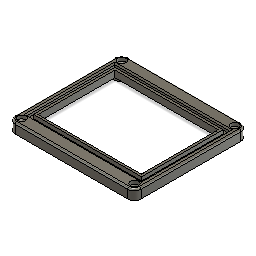
RPLIDAR Enclosure Lid (Bottom) v4 (Autodesk Fusion 360 design; units mm, degrees)
Autodesk Fusion 360 part; units mm, degrees
note: some values were not read from the file. Set by a fixed rule: which sketch regions a step uses.
sketch "Sketch1" plane through (0, 0, 0) normal (0, 1, 0) x (1, 0, 0)
  circle A0 centre (114.1757, 101.981) radius 2.032
  arc A1 (120.4909, 101.6166) -> (114.1409, 107.9666) centre (114.1409, 101.6166) ccw
  circle A2 centre (6.2257, 101.981) radius 2.032
  arc A3 (6.4449, 107.9666) -> (0.0949, 101.6166) centre (6.4449, 101.6166) ccw
  arc A4 (114.1409, -0.2374) -> (120.4909, 6.1126) centre (114.1409, 6.1126) ccw
  circle A5 centre (114.1663, 6.2142) radius 2.032
  circle A6 centre (6.2163, 6.2142) radius 2.032
  line L0 (6.4449, -0.2374) -> (114.1409, -0.2374)
  line L1 (0.0949, 101.6166) -> (0.0949, 6.1126)
  arc A7 (0.0949, 6.1126) -> (6.4449, -0.2374) centre (6.4449, 6.1126) ccw
  line L2 (114.1409, 107.9666) -> (6.4449, 107.9666)
  line L3 (120.4909, 6.1126) -> (120.4909, 101.6166)
  arc A8 (13.9701, 6.3611) -> (16.51, 3.8211) centre (16.51, 6.3611) ccw
  line L4 (103.8887, 3.8211) -> (16.51, 3.8211)
  arc A9 (103.8887, 3.8211) -> (106.4287, 6.3611) centre (103.8887, 6.3611) ccw
  line L5 (106.4287, 6.3611) -> (106.4287, 8.382)
  arc A10 (112.0167, 13.97) -> (106.4287, 8.382) centre (112.0167, 8.382) ccw
  line L6 (112.0167, 13.97) -> (114.0376, 13.97)
  arc A11 (114.0376, 13.97) -> (116.5776, 16.51) centre (114.0376, 16.51) ccw
  line L7 (116.5776, 16.51) -> (116.5776, 91.694)
  arc A12 (116.5776, 91.694) -> (114.0376, 94.234) centre (114.0376, 91.694) ccw
  line L8 (112.0167, 94.234) -> (114.0376, 94.234)
  arc A13 (106.4287, 99.822) -> (112.0167, 94.234) centre (112.0167, 99.822) ccw
  line L9 (106.4287, 101.8429) -> (106.4287, 99.822)
  arc A14 (106.4287, 101.8429) -> (103.8887, 104.3829) centre (103.8887, 101.8429) ccw
  line L10 (103.8887, 104.3829) -> (16.5127, 104.3829)
  arc A15 (16.5127, 104.3829) -> (13.9727, 101.8429) centre (16.5127, 101.8429) ccw
  line L11 (13.9727, 101.8429) -> (13.9727, 99.822)
  arc A16 (8.3847, 94.234) -> (13.9727, 99.822) centre (8.3847, 99.822) ccw
  line L12 (8.3847, 94.234) -> (6.3638, 94.234)
  arc A17 (6.3638, 94.234) -> (3.8238, 91.694) centre (6.3638, 91.694) ccw
  line L13 (3.8238, 91.694) -> (3.8238, 16.5092)
  arc A18 (3.8238, 16.5092) -> (6.3624, 13.9706) centre (6.3624, 16.5092) ccw
  line L14 (8.3818, 13.9706) -> (6.3624, 13.9706)
  arc A19 (13.9701, 8.382) -> (8.3818, 13.9706) centre (8.3818, 8.3824) ccw
  line L15 (13.9701, 6.3611) -> (13.9701, 8.382)
  line L16 (6.4422, 8.223) -> (6.5225, 8.223)
  line L17 (113.859, 8.2229) -> (110.7148, 8.2229)
  circle A20 centre (6.2163, 6.2142) radius 3.81
  circle A21 centre (114.1663, 6.2142) radius 3.81
  circle A22 centre (114.1757, 101.981) radius 3.81
  circle A23 centre (6.2257, 101.981) radius 3.81
  line L18 (8.3818, 11.8116) -> (6.3624, 11.8116)
  arc A24 (1.6648, 16.5092) -> (6.3624, 11.8116) centre (6.3624, 16.5092) ccw
  line L19 (1.6648, 91.694) -> (1.6648, 16.5092)
  arc A25 (6.3638, 96.393) -> (1.6648, 91.694) centre (6.3638, 91.694) ccw
  line L20 (8.3847, 96.393) -> (6.3638, 96.393)
  arc A26 (8.3847, 96.393) -> (11.8137, 99.822) centre (8.3847, 99.822) ccw
  line L21 (11.8137, 101.8429) -> (11.8137, 99.822)
  arc A27 (16.5127, 106.5419) -> (11.8137, 101.8429) centre (16.5127, 101.8429) ccw
  line L22 (103.8887, 106.5419) -> (16.5127, 106.5419)
  arc A28 (108.5877, 101.8429) -> (103.8887, 106.5419) centre (103.8887, 101.8429) ccw
  line L23 (108.5877, 101.8429) -> (108.5877, 99.822)
  arc A29 (108.5877, 99.822) -> (112.0167, 96.393) centre (112.0167, 99.822) ccw
  line L24 (112.0167, 96.393) -> (114.0376, 96.393)
  arc A30 (118.7366, 91.694) -> (114.0376, 96.393) centre (114.0376, 91.694) ccw
  line L25 (118.7366, 16.51) -> (118.7366, 91.694)
  arc A31 (114.0376, 11.811) -> (118.7366, 16.51) centre (114.0376, 16.51) ccw
  line L26 (112.0167, 11.811) -> (114.0376, 11.811)
  arc A32 (112.0167, 11.811) -> (108.5877, 8.382) centre (112.0167, 8.382) ccw
  line L27 (108.5877, 6.3611) -> (108.5877, 8.382)
  arc A33 (103.8887, 1.6621) -> (108.5877, 6.3611) centre (103.8887, 6.3611) ccw
  line L28 (103.8887, 1.6621) -> (16.51, 1.6621)
  arc A34 (11.8111, 6.3611) -> (16.51, 1.6621) centre (16.51, 6.3611) ccw
  line L29 (11.8111, 6.3611) -> (11.8111, 8.3822)
  arc A35 (11.8111, 8.3822) -> (8.3818, 11.8116) centre (8.3818, 8.3824) ccw
  line L30 (8.3818, 16.5106) -> (6.3638, 16.5106)
  line L31 (6.3638, 91.694) -> (6.3638, 16.5106)
  line L32 (8.3847, 91.694) -> (6.3638, 91.694)
  arc A36 (8.3847, 91.694) -> (16.5127, 99.822) centre (8.3847, 99.822) ccw
  line L33 (16.5127, 101.8429) -> (16.5127, 99.822)
  line L34 (103.8887, 101.8429) -> (16.5127, 101.8429)
  line L35 (103.8887, 101.8429) -> (103.8887, 99.822)
  arc A37 (103.8887, 99.822) -> (112.0167, 91.694) centre (112.0167, 99.822) ccw
  line L36 (112.0167, 91.694) -> (114.0376, 91.694)
  line L37 (114.0376, 16.51) -> (114.0376, 91.694)
  line L38 (112.0167, 16.51) -> (114.0376, 16.51)
  arc A38 (112.0167, 16.51) -> (103.8887, 8.382) centre (112.0167, 8.382) ccw
  line L39 (103.8887, 6.3611) -> (103.8887, 8.382)
  line L40 (103.8887, 6.3611) -> (16.5101, 6.3611)
  line L41 (16.5101, 6.3611) -> (16.5101, 8.3821)
  arc A39 (16.5101, 8.3821) -> (8.3818, 16.5106) centre (8.3818, 8.3824) ccw
  arc A40 (14.2291, 6.3611) -> (16.51, 4.0801) centre (16.51, 6.3611) ccw
  line L42 (103.8887, 4.0801) -> (16.51, 4.0801)
  arc A41 (103.8887, 4.0801) -> (106.1697, 6.3611) centre (103.8887, 6.3611) ccw
  line L43 (106.1697, 6.3611) -> (106.1697, 8.382)
  arc A42 (112.0167, 14.2291) -> (106.1697, 8.382) centre (112.0167, 8.382) ccw
  line L44 (112.0167, 14.2291) -> (114.0376, 14.2291)
  arc A43 (114.0376, 14.2291) -> (116.3186, 16.51) centre (114.0376, 16.51) ccw
  line L45 (116.3186, 16.51) -> (116.3186, 91.694)
  arc A44 (116.3186, 91.694) -> (114.0376, 93.975) centre (114.0376, 91.694) ccw
  line L46 (112.0167, 93.975) -> (114.0376, 93.975)
  arc A45 (106.1697, 99.822) -> (112.0167, 93.975) centre (112.0167, 99.822) ccw
  line L47 (106.1697, 101.8429) -> (106.1697, 99.822)
  arc A46 (106.1697, 101.8429) -> (103.8887, 104.1239) centre (103.8887, 101.8429) ccw
  line L48 (103.8887, 104.1239) -> (16.5127, 104.1239)
  arc A47 (16.5127, 104.1239) -> (14.2317, 101.8429) centre (16.5127, 101.8429) ccw
  line L49 (14.2317, 101.8429) -> (14.2317, 99.822)
  arc A48 (8.3847, 93.9749) -> (14.2317, 99.822) centre (8.3847, 99.822) ccw
  line L50 (8.3847, 93.9749) -> (6.3638, 93.9749)
  arc A49 (6.3638, 93.9749) -> (4.0828, 91.694) centre (6.3638, 91.694) ccw
  line L51 (4.0828, 91.694) -> (4.0828, 16.5092)
  arc A50 (4.0828, 16.5092) -> (6.3624, 14.2296) centre (6.3624, 16.5092) ccw
  line L52 (8.3818, 14.2296) -> (6.3624, 14.2296)
  arc A51 (14.2291, 8.3826) -> (8.3818, 14.2296) centre (8.3818, 8.3824) ccw
  line L53 (14.2291, 6.3611) -> (14.2291, 8.3826)
  arc A52 (11.6079, 6.3611) -> (16.51, 1.4589) centre (16.51, 6.3611) ccw
  line L54 (103.8887, 1.4589) -> (16.51, 1.4589)
  arc A53 (103.8887, 1.4589) -> (108.7909, 6.3611) centre (103.8887, 6.3611) ccw
  line L55 (108.7909, 6.3611) -> (108.7909, 8.382)
  arc A54 (112.0167, 11.6078) -> (108.7909, 8.382) centre (112.0167, 8.382) ccw
  line L56 (112.0167, 11.6078) -> (114.0376, 11.6078)
  arc A55 (114.0376, 11.6078) -> (118.9398, 16.51) centre (114.0376, 16.51) ccw
  line L57 (118.9398, 16.51) -> (118.9398, 91.694)
  arc A56 (118.9398, 91.694) -> (114.0376, 96.5962) centre (114.0376, 91.694) ccw
  line L58 (112.0167, 96.5962) -> (114.0376, 96.5962)
  arc A57 (108.7909, 99.822) -> (112.0167, 96.5962) centre (112.0167, 99.822) ccw
  line L59 (108.7909, 101.8429) -> (108.7909, 99.822)
  arc A58 (108.7909, 101.8429) -> (103.8887, 106.7451) centre (103.8887, 101.8429) ccw
  line L60 (103.8887, 106.7451) -> (16.5127, 106.7451)
  arc A59 (16.5127, 106.7451) -> (11.6105, 101.8429) centre (16.5127, 101.8429) ccw
  line L61 (11.6105, 101.8429) -> (11.6105, 99.822)
  arc A60 (8.3847, 96.5962) -> (11.6105, 99.822) centre (8.3847, 99.822) ccw
  line L62 (8.3847, 96.5962) -> (6.3638, 96.5962)
  arc A61 (6.3638, 96.5962) -> (1.4616, 91.694) centre (6.3638, 91.694) ccw
  line L63 (1.4616, 91.694) -> (1.4616, 16.5092)
  arc A62 (1.4616, 16.5092) -> (6.3624, 11.6084) centre (6.3624, 16.5092) ccw
  line L64 (8.3818, 11.6084) -> (6.3624, 11.6084)
  arc A63 (11.6079, 8.3825) -> (8.3818, 11.6084) centre (8.3818, 8.3824) ccw
  line L65 (11.6079, 6.3611) -> (11.6079, 8.3825)
  point P0 (16.51, 4.3291)
  point P1 (100.33, 4.3291)
  point P2 (0.0949, -0.2374)
  point P3 (120.4909, -0.2374)
  point P4 (0.0949, 107.9666)
  dimension "d1" = 4.064
  dimension "d2" = 4.064
  dimension "d3" = 4.064
  dimension "d4" = 4.064
  dimension "d11" = 120.396
  dimension "d12" = 108.204
  dimension "d13" = 6.35
  dimension "d14" = 6.35
  dimension "d15" = 6.35
  dimension "d16" = 6.35
  dimension "d58" = 7.62
  dimension "d59" = 7.62
  dimension "d60" = 7.62
  dimension "d61" = 7.62
  dimension "d141" = 5.9856
  dimension "d142" = 6.1308
  dimension "d143" = 5.588
  dimension "d144" = 2.54
  dimension "d145" = 2.54
  dimension "d146" = 13.8778
  dimension "d147" = 13.7326
  dimension "d148" = 3.5837
  dimension "d149" = 2.54
  dimension "d150" = 5.588
  dimension "d151" = 2.54
  dimension "d152" = 13.7326
  dimension "d153" = 14.0622
  dimension "d154" = 5.9856
  dimension "d155" = 6.3152
  dimension "d156" = 14.0622
  dimension "d157" = 3.9133
  dimension "d158" = 6.3246
  dimension "d159" = 3.7289
  dimension "d160" = 2.54
  dimension "d161" = 2.54
  dimension "d162" = 5.588
  dimension "d163" = 14.2074
  dimension "d164" = 6.4516
  dimension "d165" = 2.159
  dimension "d166" = 2.54
  dimension "d169" = 4.572
  dimension "d170" = 4.572
  dimension "d171" = 3.556
  dimension "d182" = 6.4516
  dimension "d183" = 6.1214
  dimension "d184" = 14.208
  dimension "d185" = 13.8752
  dimension "d205" = 0.259
  dimension "d208" = -2.3622
  constraint horizontal L0
  constraint vertical L3
  constraint horizontal L2
  constraint vertical L1
  constraint coincident P4 L2
  constraint coincident P4 L1
  constraint tangent A3 L2
  constraint tangent A3 L1
  constraint tangent A1 L3
  constraint tangent A1 L2
  constraint coincident P3 L0
  constraint coincident P3 L3
  constraint tangent A4 L0
  constraint tangent A4 L3
  constraint coincident P2 L0
  constraint coincident P2 L1
  constraint tangent L0 A7
  constraint tangent L1 A7
  constraint tangent A11 L7
  constraint tangent A9 L5
  constraint tangent L6 A11
  constraint tangent L4 A9
  constraint tangent L5 A10
  constraint tangent A10 L6
  constraint tangent A12 L8
  constraint tangent L8 A13
  constraint tangent A13 L9
  constraint tangent L13 A18
  constraint tangent L9 A14
  constraint tangent A14 L10
  constraint tangent L10 A15
  constraint tangent A16 L12
  constraint tangent L12 A17
  constraint tangent A17 L13
  constraint tangent A18 L14
  constraint tangent L14 A19
  constraint parallel L0 L16
  constraint coincident A6 L16.end
  constraint coincident A5 L17.start
  constraint concentric A6 A20
  constraint concentric A5 A21
  constraint concentric A0 A22
  constraint concentric A2 A23
  measures "d1" diameter of A2
  measures "d2" diameter of A0
  measures "d3" diameter of A5
  measures "d4" diameter of A6
  measures "d11" distance of P2 P3
  measures "d12" distance of P2 P4
  measures "d13" radius of A3
  measures "d14" radius of A1
  measures "d15" radius of A4
  measures "d16" radius of A7
  measures "d58" diameter of A20
  measures "d59" diameter of A21
  measures "d60" diameter of A22
  measures "d61" diameter of A23
  measures "d141" vertical distance of A3.start A2.centre
  measures "d142" horizontal distance of A3.end A2.centre
  measures "d143" radius of A16
  measures "d144" radius of A15
  measures "d145" radius of A17
  measures "d146" distance of L1 L11
  measures "d147" distance of L2 L12
  measures "d148" distance of L2 L10
  measures "d149" radius of A14
  measures "d150" radius of A13
  measures "d151" radius of A12
  measures "d152" distance of L2 L8
  measures "d153" distance of L3 L9
  measures "d154" vertical distance of A1.end A0.centre
  measures "d155" horizontal distance of A1.start A0.centre
  measures "d156" distance of L3 L5
  measures "d157" distance of L3 L7
  measures "d158" horizontal distance of A5.centre A4.end
  measures "d159" distance of L1 L13
  measures "d160" radius of A11
  measures "d161" radius of A9
  measures "d162" radius of A10
  measures "d163" distance of L0 L6
  measures "d164" vertical distance of A5.centre A4.start
  measures "d182" distance of A6.centre L0
  measures "d183" distance of A6.centre L1
  measures "d184" distance of L0 L14
  measures "d185" distance of L1 L15
extrude "Extrude1" add sketch "Sketch1" along normal blind 9.652 contours A1 A3 A4 L0 L1 A7 L2 L3 | A8 L4 A9 L5 A10 L6 A11 L7 A12 L8 A13 L9 A14 L10 A15 L11 A16 L12 A17 L13 A18 L14 A19 L15 | A20 | A21 | A22 | A23 | L18 A24 L19 A25 L20 A26 L21 A27 L22 A28 L23 A29 L24 A30 L25 A31 L26 A32 L27 A33 L28 A34 L29 A35 | L30 L31 L32 A36 L33 L34 L35 A37 L36 L37 L38 A38 L39 L40 L41 A39 | A40 L42 A41 L43 A42 L44 A43 L45 A44 L46 A45 L47 A46 L48 A47 L49 A48 L50 A49 L51 A50 L52 A51 L53 | A52 L54 A53 L55 A54 L56 A55 L57 A56 L58 A57 L59 A58 L60 A59 L61 A60 L62 A61 L63 A62 L64 A63 L65
sketch "Sketch2" plane through (0, 9.652, 0) normal (0, 1, 0) x (-1, 0, 0)
  circle A0 centre (-114.1663, -6.2142) radius 2.032
  circle A1 centre (-6.2257, -101.981) radius 2.032
  circle A2 centre (-6.2163, -6.2142) radius 2.032
  circle A3 centre (-114.1757, -101.981) radius 2.032
  line L0 (-120.4909, -6.1126) -> (-120.4909, -101.6166)
  arc A4 (-120.4909, -101.6166) -> (-114.1409, -107.9666) centre (-114.1409, -101.6166) ccw
  line L1 (-114.1409, -107.9666) -> (-6.4449, -107.9666)
  arc A5 (-6.4449, -107.9666) -> (-0.0949, -101.6166) centre (-6.4449, -101.6166) ccw
  line L2 (-0.0949, -101.6166) -> (-0.0949, -6.1126)
  arc A6 (-0.0949, -6.1126) -> (-6.4449, 0.2374) centre (-6.4449, -6.1126) ccw
  line L3 (-6.4449, 0.2374) -> (-114.1409, 0.2374)
  arc A7 (-114.1409, 0.2374) -> (-120.4909, -6.1126) centre (-114.1409, -6.1126) ccw
  circle A8 centre (-6.2163, -6.2142) radius 3.81
  circle A9 centre (-114.1663, -6.2142) radius 3.81
  circle A10 centre (-114.1757, -101.981) radius 3.81
  circle A11 centre (-6.2257, -101.981) radius 3.81
  dimension "d123" = 5.9436
  dimension "d186" = 6.4516
  dimension "d187" = 6.3246
  dimension "d212" = 7.62
  dimension "d213" = 7.62
  dimension "d214" = 7.62
  dimension "d215" = 7.62
  constraint concentric A3 A10
  constraint concentric A1 A11
  measures "d186" distance of L3 A0.centre
  measures "d187" distance of L0 A0.centre
  measures "d212" diameter of A10
  measures "d213" diameter of A11
  measures "d214" diameter of A8
  measures "d215" diameter of A9
extrude "Extrude9" cut sketch "Sketch2" against normal blind 3.175 contours A11
chamfer "Chamfer1" distance 2.0574 distance2 1.778 1 edges at (4.3312, 6.477, -101.2462) measured on face at (8.2476, 4.318, -102.1833)
extrude "Extrude10" cut sketch "Sketch2" against normal blind 3.175 contours A10
extrude "Extrude11" cut sketch "Sketch2" against normal blind 3.175 contours A9
extrude "Extrude12" cut sketch "Sketch2" against normal blind 3.175 contours A8
chamfer "Chamfer2" distance 2.0574 distance2 1.778 1 edges at (112.2812, 6.477, -101.2462) measured on face at (116.1976, 4.318, -102.1833)
chamfer "Chamfer3" distance 2.0574 distance2 1.778 1 edges at (112.2718, 6.477, -5.4794) measured on face at (116.1882, 4.318, -6.4165)
chamfer "Chamfer4" distance 2.0574 distance2 1.778 1 edges at (4.3218, 6.477, -5.4794) measured on face at (8.2382, 4.318, -6.4165)
extrude "Extrude13" cut sketch "Sketch1" along normal blind 3.048 contours L18 A24 L19 A25 L20 A26 L21 A27 L22 A28 L23 A29 L24 A30 L25 A31 L26 A32 L27 A33 L28 A34 L29 A35
extrude "Extrude14" cut sketch "Sketch1" along normal blind 3.302 contours L30 L31 L32 A36 L33 L34 L35 A37 L36 L37 L38 A38 L39 L40 L41 A39
sketch "Sketch3" plane through (0, 9.652, 0) normal (0, 1, 0) x (-1, 0, 0)
  circle A0 centre (-6.2163, -6.2142) radius 3.81
  circle A1 centre (-114.1663, -6.2142) radius 3.81
  circle A2 centre (-114.1757, -101.981) radius 3.81
  circle A3 centre (-6.2257, -101.981) radius 3.81
  line L0 (-120.4909, -6.1126) -> (-120.4909, -101.6166)
  arc A4 (-120.4909, -101.6166) -> (-114.1409, -107.9666) centre (-114.1409, -101.6166) ccw
  line L1 (-114.1409, -107.9666) -> (-6.4449, -107.9666)
  arc A5 (-6.4449, -107.9666) -> (-0.0949, -101.6166) centre (-6.4449, -101.6166) ccw
  line L2 (-0.0949, -101.6166) -> (-0.0949, -6.1126)
  arc A6 (-0.0949, -6.1126) -> (-6.4449, 0.2374) centre (-6.4449, -6.1126) ccw
  line L3 (-6.4449, 0.2374) -> (-114.1409, 0.2374)
  arc A7 (-114.1409, 0.2374) -> (-120.4909, -6.1126) centre (-114.1409, -6.1126) ccw
  line L4 (-5.4289, -96.2826) -> (-115.1569, -96.2826)
  line L5 (-115.1569, -96.2826) -> (-115.1569, -11.9546)
  line L6 (-115.1569, -11.9546) -> (-5.4289, -11.9546)
  line L7 (-5.4289, -11.9546) -> (-5.4289, -96.2826)
  line L8 (-111.9819, -93.1076) -> (-111.9819, -15.1296)
  line L9 (-111.9819, -15.1296) -> (-8.6039, -15.1296)
  line L10 (-8.6039, -15.1296) -> (-8.6039, -93.1076)
  line L11 (-8.6039, -93.1076) -> (-111.9819, -93.1076)
  line L12 (-109.5689, -90.8216) -> (-109.5689, -17.0346)
  line L13 (-10.8899, -17.0346) -> (-10.8899, -90.8216)
  line L14 (-10.8899, -90.8216) -> (-109.5689, -90.8216)
  line L15 (-10.8899, -90.8216) -> (-109.6959, -90.8216)
  line L16 (-109.6959, -90.8216) -> (-109.6959, -17.1616)
  line L17 (-109.6959, -17.1616) -> (-10.8899, -17.1616)
  line L18 (-10.8899, -17.1616) -> (-10.8899, -90.8216)
  dimension "d174" = 5.334
  dimension "d175" = 5.334
  dimension "d176" = 11.684
  dimension "d177" = 12.192
  dimension "d178" = 3.175
  dimension "d188" = 2.286
  dimension "d189" = 2.032
  dimension "d190" = 2.286
  dimension "d191" = 2.286
  constraint horizontal L4
  constraint vertical L5
  constraint horizontal L6
  constraint vertical L7
  constraint horizontal L15
  constraint vertical L16
  constraint horizontal L17
  constraint vertical L18
  constraint parallel L5 L12
  constraint parallel L7 L13
  constraint parallel L4 L14
  measures "d174" distance of L0 L5
  measures "d175" distance of L2 L7
  measures "d176" distance of L1 L4
  measures "d177" distance of L3 L6
  measures "d188" distance of L11 L15
  measures "d189" distance of L9 L17
  measures "d190" distance of L10 L18
  measures "d191" distance of L8 L16
extrude "Extrude16" cut sketch "Sketch3" against normal blind 3.556 contours L4 L5 L6 L7
extrude "Extrude17" cut sketch "Sketch3" against normal blind 10.16 contours L12 L15 L16 L17 | L12 L13 L14 L15 L17 L18
fillet "Fillet1" radius 2.032 1 edges at (109.6959, 6.477, -90.8216)
fillet "Fillet2" radius 2.032 1 edges at (109.6959, 6.477, -17.1616)
fillet "Fillet3" radius 2.032 1 edges at (10.8899, 6.477, -17.1616)
fillet "Fillet4" radius 2.032 1 edges at (10.8899, 6.477, -90.8216)
fillet "Fillet5" radius 1.651 8 edges at (120.4909, 9.652, -53.8646) (118.631, 9.652, -106.1067) (60.2929, 9.652, -107.9666) (1.9547, 9.652, -106.1067) (0.0949, 9.652, -53.8646) (1.9547, 9.652, -1.6225) (60.2929, 9.652, 0.2374) (118.631, 9.652, -1.6225)
extrude "Extrude15" cut sketch "Sketch3" against normal blind 10.16 contours L12 L13 L14 L15 L17 L18
sketch "Sketch4" plane through (0, 3.302, 0) normal (0, -1, 0) x (1, 0, 0)
  line L0 (103.8887, -8.382) -> (103.8887, -6.3611)
  line L1 (103.8887, -6.3611) -> (16.5101, -6.3611)
  line L2 (16.5101, -6.3611) -> (16.5101, -8.3821)
  arc A0 (8.3818, -16.5106) -> (16.5101, -8.3821) centre (8.3818, -8.3824) ccw
  line L3 (8.3818, -16.5106) -> (6.3638, -16.5106)
  line L4 (6.3638, -16.5106) -> (6.3638, -91.694)
  line L5 (6.3638, -91.694) -> (8.3847, -91.694)
  arc A1 (16.5127, -99.822) -> (8.3847, -91.694) centre (8.3847, -99.822) ccw
  line L6 (16.5127, -99.822) -> (16.5127, -101.8429)
  line L7 (16.5127, -101.8429) -> (103.8887, -101.8429)
  line L8 (103.8887, -101.8429) -> (103.8887, -99.822)
  arc A2 (112.0167, -91.694) -> (103.8887, -99.822) centre (112.0167, -99.822) ccw
  line L9 (112.0167, -91.694) -> (114.0376, -91.694)
  line L10 (114.0376, -91.694) -> (114.0376, -16.51)
  line L11 (114.0376, -16.51) -> (112.0167, -16.51)
  arc A3 (103.8887, -8.382) -> (112.0167, -16.51) centre (112.0167, -8.382) ccw
  line L12 (109.5689, -90.8216) -> (10.8899, -90.8216)
  line L13 (10.8899, -90.8216) -> (10.8899, -17.1616)
  line L14 (10.8899, -17.1616) -> (109.5689, -17.1616)
  line L15 (109.6959, -19.1936) -> (109.6959, -88.7896)
  arc A4 (25.2774, -41.6726) -> (25.2774, -67.0726) centre (25.2774, -54.3726) ccw
  line L16 (6.4449, 0.2374) -> (114.1409, 0.2374)
  line L17 (109.5689, -89.4967) -> (109.5689, -90.8216)
  line L18 (109.5689, -17.1616) -> (109.5689, -18.4865)
  arc A5 (109.6959, -19.1936) -> (109.5689, -18.4865) centre (107.6639, -19.1936) ccw
  arc A6 (109.5689, -89.4967) -> (109.6959, -88.7896) centre (107.6639, -88.7896) ccw
  dimension "d201" = 54.61
  dimension "d202" = 12.7
  measures "d201" distance of A4.centre L16
  measures "d202" radius of A4
extrude "Extrude19" cut sketch "Sketch1" along normal blind 3.048 contours A8 L4 A9 L5 A10 L6 A11 L7 A12 L8 A13 L9 A14 L10 A15 L11 A16 L12 A17 L13 A18 L14 A19 L15
extrude "Extrude20" cut sketch "Sketch1" along normal blind 3.048 contours A52 L54 A53 L55 A54 L56 A55 L57 A56 L58 A57 L59 A58 L60 A59 L61 A60 L62 A61 L63 A62 L64 A63 L65
chamfer "Chamfer5" distance 1.2192 angle 45 4 edges at (60.2929, 9.652, -11.9546) (115.1569, 9.652, -54.1186) (60.2929, 9.652, -96.2826) (5.4289, 9.652, -54.1186)
